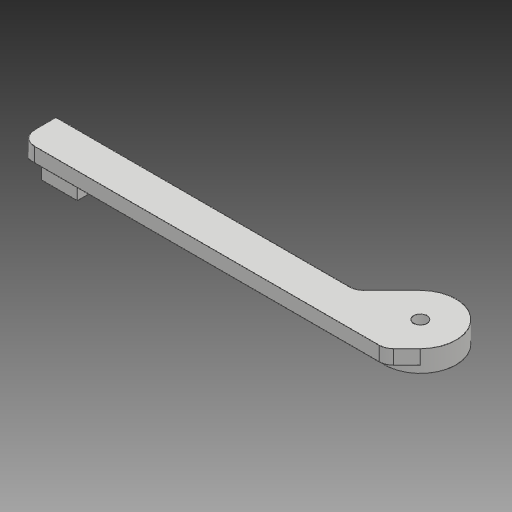
# Autodesk Inventor part: Akkusperre
Saved by Autodesk Inventor 2019.4 (Build 234330000, 330)
## iProperties
Part Number: Akkusperre
Material: Generisch
Document SubType Name: Modeling
Designer: rYan
Density: 1 g/cm^3
Appearance: Vorgabe
Mass: 0.782953 g
Surface Area: 10.3011 cm^2
Volume: 0.782953 cm^3
Author: rYan
Autodesk Inventor part; units mm, degrees
ref_plane "YZ Plane" through (0, 0, 0) normal (1, 0, 0) x (0, 1, 0)
ref_plane "XZ Plane" through (0, 0, 0) normal (0, 1, 0) x (-1, 0, 0)
ref_plane "XY Plane" through (0, 0, 0) normal (0, 0, 1) x (1, 0, 0)
sketch "Skizze1" plane through (0, 0, 0) normal (0, 0, 1) x (1, 0, 0)
  line L0 (0, 9.6853) -> (0, -8.6142) projected
  line L1 (-61.4142, 0) -> (18.4853, 0) projected
  arc A0 (3.5355, -3.5355) -> (-3.5355, 3.5355) centre (0, 0) ccw
  line L2 (-8.0711, -1) -> (-50, -1)
  line L3 (-50, -1) -> (-50, -6)
  line L4 (-50, -6) -> (1.0711, -6)
  line L5 (3.5355, -3.5355) -> (1.0711, -6)
  line L6 (-8.0711, -1) -> (-3.5355, 3.5355)
  dimension "d1" = 5
  dimension "d2" = 1
  dimension "d3" = 5
  dimension "d21" = 50
  dimension "d22" = 45
  constraints: 10 end point, 2 perpendicular, 2 point on circle, 2 tangent, 1 centre point, 1 coincident, 1 parallel
  measures "d1" radius of A0
  measures "d2" distance between parallel lines of L2 L1
  measures "d3" distance of L2.end L3.end
  measures "d21" distance between parallel lines of L3 L0
  measures "d22" angle of L6 L2
extrude "Extrusion1" add sketch "Skizze1" along normal blind 2
sketch "Skizze2" plane through (0, 0, 0) normal (0, 0, 1) x (1, 0, 0)
  point P0 (0, 0)
  point P1 (0, 0)
  constraints: 1 coincident
hole "Bohrung1" at (0, 0, 0) direction (0, 0, 1) diameter 1.9 end through all
sketch "Skizze5" plane through (-50, -6, 0) normal (-1, 0, 0) x (0, 0, 1)
  line L0 (0, 5) -> (0, 0) projected
  line L1 (0, 0) -> (2, 0) projected
  line L2 (2, 5) -> (2, 0) projected
  line L3 (0, 5) -> (2, 5) projected
  line L4 (0, 0) -> (2, 0) projected
  line L5 (0, 0) -> (-2, 2.3835)
  line L6 (-2, 2.3835) -> (-2, 3)
  line L7 (0, 5) -> (0, 0) projected
  line L8 (0, 0) -> (0, 5)
  line L9 (-2, 3) -> (-4.6, 3)
  line L10 (-4.6, 3) -> (-4.6, 5)
  line L11 (-4.6, 5) -> (0, 5)
  point P0 (0, 6)
  dimension "d23" = 40
  dimension "d28" = 3
  dimension "d29" = 2
  dimension "d30" = 4.6
  constraints: 12 end point, 3 perpendicular, 1 collinear, 1 horizontal
  measures "d23" angle of L0 L5
  measures "d28" distance between parallel lines of L1 L9
  measures "d29" distance between parallel lines of L0 L6
  measures "d30" distance between parallel lines of L0 L10
extrude "Extrusion4" add sketch "Skizze5" against normal blind 5 contours L0 L5 L6 L9 L10 L11
fillet "Rundung1" radius 2 3 edges at (1.0711, -6, 1) (-8.0711, -1, 1) (-50, -6, 1)
sketch "Skizze8" plane through (0, 0, 0) normal (0, 0, -1) x (-1, 0, 0)
  circle A0 centre (0, 0) radius 5
  arc A1 (3.5355, 3.5355) -> (-3.5355, -3.5355) centre (0, 0) ccw projected
  circle A2 centre (0, 0) radius 0.95 projected
  constraints: 1 centre point, 1 coincident, 1 concentric
extrude "Extrusion7" add sketch "Skizze8" along normal blind 1
sketch "Skizze6" plane through (0, 0, -1) normal (0, 0, -1) x (-1, 0, 0)
  circle A0 centre (0, 0) radius 1.5
  circle A1 centre (0, 0) radius 0.95 projected
  circle A2 centre (0, 0) radius 0.95 projected
  dimension "d32" = 3
  constraints: 1 centre point, 1 coincident
  measures "d32" diameter of A0
extrude "Extrusion5" add sketch "Skizze6" along normal blind 2.2
sketch "Skizze7" plane through (0, 0, -3.2) normal (0, 0, -1) x (-1, 0, 0)
  line L0 (0.2, 2) -> (-0.2, 2)
  line L1 (-0.2, 2) -> (-0.2, -2)
  line L2 (-0.2, -2) -> (0.2, -2)
  line L3 (0.2, -2) -> (0.2, 2)
  line L4 (0.2, 2) -> (-0.2, -2) construction
  line L5 (-0.2, 2) -> (0.2, -2) construction
  point P0 (0, 0)
  dimension "d35" = 0.4
  dimension "d36" = 4
  constraints: 12 end point, 2 midpoint, 2 parallel, 1 horizontal, 1 perpendicular
  measures "d35" distance of L2.end L1.end
  measures "d36" distance of L1.end L0.end
extrude "Extrusion6" cut sketch "Skizze7" against normal up to surface (2.2 mm away)
